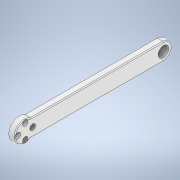
# Autodesk Inventor part: base5
Saved by Autodesk Inventor 2022 (Build 260153000, 153)
## iProperties
Created: 2022-06-14
Part Number: base5
Material: ABS プラスチック
Document SubType Name: Modeling
Designer: yuto6
Density: 1.06 g/cm^3
Appearance: 滑らか - 白
Author: yuto6
Autodesk Inventor part; units mm, degrees
ref_plane "YZ Plane" through (0, 0, 0) normal (1, 0, 0) x (0, 1, 0)
ref_plane "XZ Plane" through (0, 0, 0) normal (0, 1, 0) x (-1, 0, 0)
ref_plane "XY Plane" through (0, 0, 0) normal (0, 0, 1) x (1, 0, 0)
sketch "スケッチ1" plane through (0, 0, 0) normal (1, 0, 0) x (0, 1, 0)
  circle A0 centre (0, 0) radius 12
  line L0 (0, 0) -> (10, 0)
  line L1 (10, 0) -> (10, -170)
  line L2 (10, -170) -> (0, -170)
  line L3 (0, -170) -> (0, 0)
  point P0 (10, -6.6332)
  point P1 (0, -12)
  dimension "d0" = 24
  dimension "d1" = 170
  dimension "d2" = 10
  constraints: 8 end point, 2 parallel, 1 centre point, 1 coincident, 1 horizontal, 1 perpendicular
  measures "d0" diameter of A0
  measures "d1" distance of L0.end L1.end
  measures "d2" distance of L1.end L2.end
extrude "押し出し1" add sketch "スケッチ1" along normal blind 8 contours A0 L1 L0 L3 | L3 L0 L1 A0
sketch "スケッチ2" plane through (8, 0, 0) normal (1, 0, 0) x (0, 0, -1)
  circle A0 centre (0, 0) radius 8.5
  point P0 (0, 8.5)
  dimension "d7" = 17
  constraints: 1 coincident, 1 vertical alignment, 2 other
hole "穴1" at (8, 8.5, 0) direction (-1, 0, 0) diameter 3.4 end through all counterbore diameter 6.5 counterbore depth 3 clearance for "Socket Head Cap Screw" size "M3" standard "Ansi Metric M Profile"
pattern_circular "円形状パターン1" count 4 over 360 about axis through (0, 0, 0) along (1, 0, 0) of "穴1"
extrude "押し出し2" add sketch "スケッチ1" along normal blind 8 contours A0 L1 L2 L3
mirror "ミラー1" about plane through (0, 0, 0) normal (0, 1, 0) of "押し出し2"
sketch "スケッチ4" plane through (8, 0, 0) normal (1, 0, 0) x (0, 0, -1)
  line L0 (170, 10) -> (170, -10) projected
  point P0 (0, 0)
  point P1 (160, 0)
  dimension "d23" = 10
  measures "d23" distance from line of L0 point (160, 0)
hole "穴2" at (8, 0, -160) direction (-1, 0, 0) diameter 12.3 end through all
fillet "フィレット1" radius 10 2 edges at (4, 10, -170) (4, -10, -170)
fillet "フィレット2" radius 1 6 edges at (8, -10, -83.3169) (8, 10, -83.3169) (8, 0, 12) (0, -10, -83.3169) (0, 10, -83.3169) (0, 0, 12)
sketch "スケッチ3" plane through (8, 0, 0) normal (1, 0, 0) x (0, 0, -1)
  point P0 (0, 0)
